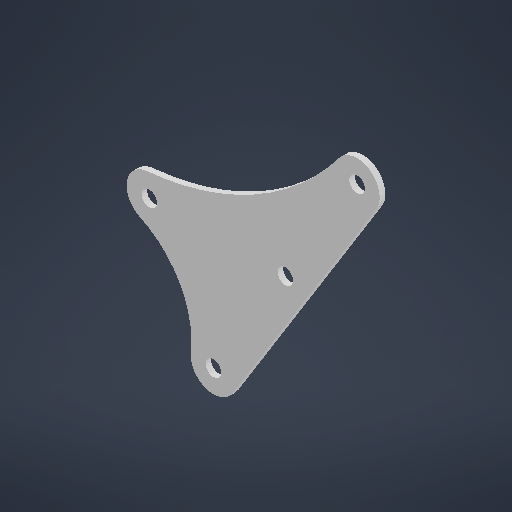
# Autodesk Inventor part: Side Poly
Saved by Autodesk Inventor 2025.1 (Build 291241000, 241)
## iProperties
Created: 2025-01-09
Part Number: Side Poly
Material: Generic
Document SubType Name: Modeling
Designer: Derek Chen
Density: 1 g/cm^3
Appearance: Default
Author: Derek Chen
Autodesk Inventor part; units mm, degrees
ref_plane "YZ Plane" through (0, 0, 0) normal (1, 0, 0) x (0, 1, 0)
ref_plane "XZ Plane" through (0, 0, 0) normal (0, 1, 0) x (-1, 0, 0)
ref_plane "XY Plane" through (0, 0, 0) normal (0, 0, 1) x (1, 0, 0)
sketch "Sketch1" plane through (0, 0, 0) normal (0, 0, 1) x (1, 0, 0)
  circle A0 centre (-74.1769, -5.2291) radius 2.1844
  circle A1 centre (-112.2444, -5.4371) radius 2.1844
  circle A2 centre (-94.297, -37.5832) radius 2.1844
  circle A3 centre (-54.0602, 27.1276) radius 2.1844
  arc A4 (-100.6091, -36.8907) -> (-114.967, -11.1738) centre (-125.8576, -34.1206) ccw
  arc A5 (-112.8432, 0.8846) -> (-59.1316, 30.942) centre (-120.0293, 76.745) ccw
  arc A6 (-112.8432, 0.8846) -> (-114.967, -11.1738) centre (-112.2444, -5.4371) ccw
  line L0 (-88.9043, -40.936) -> (-48.6711, 23.7771)
  arc A7 (-48.6711, 23.7771) -> (-59.1316, 30.942) centre (-54.0602, 27.1276) ccw
  arc A8 (-100.6091, -36.8907) -> (-88.9043, -40.936) centre (-94.297, -37.5832) ccw
  dimension "d6" = 25.4
  dimension "d8" = 76.2
  constraints: 10 point on circle, 9 centre point, 3 coincident, 2 end point
  measures "d6" radius of A4
  measures "d8" radius of A5
extrude "Extrusion3" add sketch "Sketch1" along normal blind 1.5875
body "Solid3"
